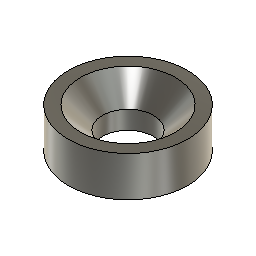
M8 Senkkopf Unterlegscheibe v2 (Autodesk Fusion 360 design; units mm, degrees)
Autodesk Fusion 360 part; units mm, degrees
sketch "Sketch1" plane through (0, 0, 0) normal (0, 1, 0) x (1, 0, 0)
  line L0 (4.2, 0) -> (9.8, 0)
  line L1 (7.8, -6.6) -> (4.2, -3)
  line L2 (4.2, -3) -> (4.2, 0)
  line L3 (7.8, -6.6) -> (9.8, -6.6)
  line L4 (9.8, -6.6) -> (9.8, 0)
  dimension "d2" = 4.2
  dimension "d3" = 9.8
  dimension "d4" = 3
  dimension "d5" = 2
  dimension "d6" = 135
  constraint horizontal L0
  constraint perpendicular L0 L2
  constraint horizontal L3
  constraint perpendicular L3 L4
  constraint coincident L0.end L4.end
  constraint horizontal origin L0.start
  measures "d2" distance of origin L0.start
  measures "d3" distance of origin L0.end
  measures "d4" distance of L0.start L1.end
  measures "d5" distance of L1.start L3.end
  measures "d6" angle of L1 L2
revolve "Revolve1" add sketch "Sketch1" angle 360 about axis through (0, 0, 1.75) along (0, 0, 1)
